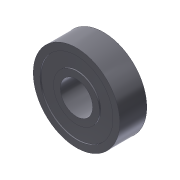
# Autodesk Inventor part: P03 - Bearing 62012
Saved by Autodesk Inventor 2016 (Build 200138000, 138)
## iProperties
Created: 2016-12-26
Part Number: P03 - Bearing 62012
Material: SAE 1020
Document SubType Name: Modeling
Designer: Fernando
Stock Number: 0
Mass: 51.6739 g
Surface Area: 29.0283 cm^2
Volume: 6.56593 cm^3
Density: 7.87 g/cm^3
Appearance: Steel - Polished
SurfaceArea_m2: 0
Author: Fernando
Autodesk Inventor part; units mm, degrees
ref_plane "YZ Plane" through (0, 0, 0) normal (1, 0, 0) x (0, 1, 0)
ref_plane "XZ Plane" through (0, 0, 0) normal (0, 1, 0) x (-1, 0, 0)
ref_plane "XY Plane" through (0, 0, 0) normal (0, 0, 1) x (1, 0, 0)
sketch "Sketch2" plane through (0, 0, 0) normal (0, 0, 1) x (1, 0, 0)
  line L0 (0, 0) -> (0, 4.9506) construction
  line L1 (-8.5, -5) -> (-6, -5)
  line L2 (-6, -5) -> (-6, 5)
  line L3 (-6, 5) -> (-8.5, 5)
  line L4 (-8.5, 5) -> (-8.5, -5)
  line L5 (-8.5, -5) -> (-6, 5) construction
  line L6 (-6, -5) -> (-8.5, 5) construction
  line L7 (-16, -5) -> (-13.5, -5)
  line L8 (-13.5, -5) -> (-13.5, 5)
  line L9 (-13.5, 5) -> (-16, 5)
  line L10 (-16, 5) -> (-16, -5)
  line L11 (-16, -5) -> (-13.5, 5) construction
  line L12 (-13.5, -5) -> (-16, 5) construction
  line L13 (-13.5, -4.5) -> (-8.5, -4.5)
  line L14 (-8.5, -4.5) -> (-8.5, 4.5)
  line L15 (-8.5, 4.5) -> (-13.5, 4.5)
  line L16 (-13.5, 4.5) -> (-13.5, -4.5)
  line L17 (-13.5, -4.5) -> (-8.5, 4.5) construction
  line L18 (-8.5, -4.5) -> (-13.5, 4.5) construction
  point P0 (-7.25, 0)
  point P1 (-14.75, 0)
  point P2 (-11, 0)
  point P3 (-14.75, 0)
  point P4 (-7.25, 0)
  dimension "d11" = 12
  dimension "d12" = 32
  dimension "d13" = 2.5
  dimension "d14" = 2.5
  dimension "d15" = 10
  dimension "d16" = 9
  constraints: 38 end point, 8 midpoint, 6 parallel, 3 horizontal, 3 horizontal alignment, 3 perpendicular, 3 point on line, 1 vertical
  measures "d11" diameter of L2 L0
  measures "d12" diameter of L10 L0
  measures "d13" distance of L8.end L9.end
  measures "d14" distance between parallel lines of L2 L14
  measures "d15" distance of L1.end L2.end
  measures "d16" distance between parallel lines of L13 L15
revolve "Revolution1" add sketch "Sketch2" angle 360 about axis through (0, 0, 0) along (0, 1, 0)
body "Solid2"
